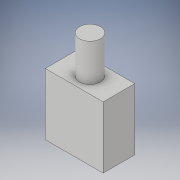
# Autodesk Inventor part: Hew Switch Box
Saved by Autodesk Inventor 2017 (Build 210142000, 142)
## iProperties
Created: 2016-09-27
Part Number: Hew Switch Box
Material: Generic
Document SubType Name: Modeling
Designer: situh
Density: 1 g/cm^3
Appearance: Default
Author: situh
Autodesk Inventor part; units mm, degrees
ref_plane "YZ Plane" through (0, 0, 0) normal (1, 0, 0) x (0, 1, 0)
ref_plane "XZ Plane" through (0, 0, 0) normal (0, 1, 0) x (-1, 0, 0)
ref_plane "XY Plane" through (0, 0, 0) normal (0, 0, 1) x (1, 0, 0)
sketch "Sketch1" plane through (0, 0, 0) normal (0, 0, 1) x (1, 0, 0)
  line L0 (-7.7703, 6.1161) -> (5.2091, 6.1161)
  line L1 (5.2091, 6.1161) -> (5.2091, -7.7269)
  line L2 (5.2091, -7.7269) -> (-7.7703, -7.7269)
  line L3 (-7.7703, -7.7269) -> (-7.7703, 6.1161)
  point P0 (0, 0)
  dimension "d0" = 12.9794
  dimension "d1" = 13.843
  constraints: 8 end point, 2 parallel, 1 horizontal, 1 perpendicular
  measures "d0" distance of L1.end L2.end
  measures "d1" distance of L2.end L0.start
extrude "Extrusion1" add sketch "Sketch1" along normal blind 7.0866
sketch "Sketch2" plane through (-7.7703, 6.1161, 0) normal (0, 1, 0) x (1, 0, 0)
  line L0 (12.9794, 0) -> (12.9794, -7.0866)
  circle A0 centre (6.4897, -3.5433) radius 2.3495
  point P0 (7.7703, 0)
  dimension "d4" = 4.699
  constraints: 2 end point, 1 centre point
  measures "d4" diameter of A0
extrude "Extrusion2" add sketch "Sketch2" along normal blind 8.4074
body "Solid1"
